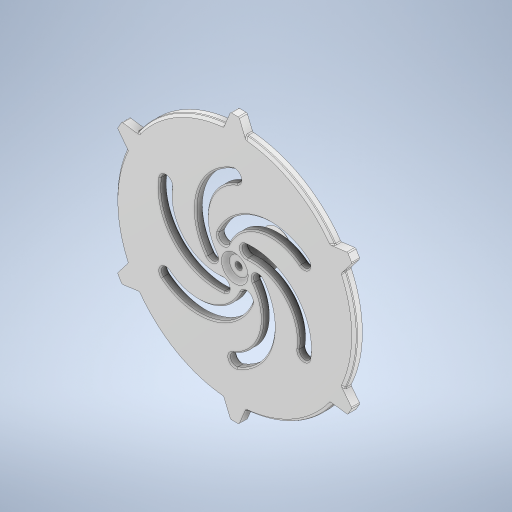
# Autodesk Inventor part: Spool Holder Iris Rotor
Saved by Autodesk Inventor 2024 (Build 280153000, 153)
## iProperties
Created: 2024-08-17
Part Number: Spool Holder Iris Rotor
Material: ABS Plastic
Document SubType Name: Modeling
Designer: Ishaan
Density: 1.06 g/cm^3
Appearance: Smooth - White
Author: Ishaan
Autodesk Inventor part; units mm, degrees
sketch "Sketch1" plane through (0, 0, 0) normal (0, 0, 1) x (1, 0, 0)
  circle A0 centre (0, 0) radius 90
  circle A1 centre (0, 0) radius 7
  dimension "d0" = 180
  dimension "d1" = 14
  constraints: 2 centre point, 2 coincident
  measures "d0" diameter of A0
  measures "d1" diameter of A1
extrude "Extrusion1" add sketch "Sketch1" against normal blind 6
sketch "Sketch2" plane through (0, 0, -6) normal (0, 0, -1) x (-1, 0, 0)
  circle A0 centre (0, 0) radius 90 projected
  circle A1 centre (0, 0) radius 7 projected
  circle A2 centre (0, 0) radius 9.9
  circle A3 centre (0, 0) radius 11
  dimension "d4" = 19.8
  dimension "d21" = 22
  constraints: 2 centre point, 2 coincident
  measures "d4" diameter of A2
  measures "d21" diameter of A3
extrude "Extrusion2" add sketch "Sketch2" along normal blind 16.4 contours A2 | A3
ref_plane "Work Plane1" through (0, 0, -26.65) normal (0, 0, -1) x (-1, 0, 0)
extrude "Extrusion3" add sketch "Sketch2" along normal up to surface (20.65 mm away) contours A2
ref_plane "Work Plane2" through (0, 0, -3) normal (0, 0, 1) x (1, 0, 0)
sketch "Sketch5" plane through (0, 0, -3) normal (0, 0, 1) x (1, 0, 0)
  circle A0 centre (0, 0) radius 7 projected
  circle A1 centre (0, 0) radius 90 projected
extrude "Extrusion6" add sketch "Sketch5" against normal up to surface (23.65 mm away) contours A0
chamfer "Chamfer8" distance 3 angle 45 1 edges at (-7, 0, 0)
chamfer "Chamfer4" distance 1 angle 45 1 edges at (11, 0, -6)
sketch "Sketch4" plane through (0, 0, 0) normal (0, 0, 1) x (1, 0, 0)
  circle A0 centre (-17.5, 0) radius 4.25 construction
  circle A1 centre (0, 0) radius 12 construction
  circle A2 centre (0, 60) radius 4.25 construction
  arc A3 (0, 60) -> (-17.5, 0) centre (14.0487, 23.3504) ccw construction
  arc A4 (-1.5212, 63.9684) -> (-20.9161, -2.5284) centre (14.0487, 23.3504) ccw
  arc A5 (1.5212, 56.0316) -> (-14.0839, 2.5284) centre (14.0487, 23.3504) ccw
  arc A6 (1.5212, 56.0316) -> (-1.5212, 63.9684) centre (0, 60) ccw
  arc A7 (-20.9161, -2.5284) -> (-14.0839, 2.5284) centre (-17.5, 0) ccw
  dimension "d32" = 8.5
  dimension "d33" = 17.5
  dimension "d35" = 60
  dimension "d36" = 35
  constraints: 10 point on circle, 7 centre point, 5 tangent, 1 equal radius, 1 horizontal alignment, 1 vertical alignment
  measures "d32" diameter of A0
  measures "d33" distance of point (0, 0) A0.centre
  measures "d35" distance of A2.centre point (0, 0)
  measures "d36" radius of A5
extrude "Extrusion5" cut sketch "Sketch4" against normal through all
pattern_circular "Circular Pattern1" count 6 over 360 about axis through (0, 0, 0) along (0, 0, -1) of "Extrusion5"
chamfer "Chamfer6" distance 2 angle 45 1 edges at (-90, 0, 0)
chamfer "Chamfer7" distance 1 angle 45 48 edges at (-38.4847, -0.3567, 0) (-4.5274, -14.6739, 0) (-44.6258, -6.2335, 0) (-51.2947, 34.1974, 0) (-38.4847, -0.3567, -6) (-51.2947, 34.1974, -6) (-44.6258, -6.2335, -6) (-4.5274, -14.6739, -6) (-18.9334, -33.5071, 0) (10.4442, -11.2577, 0) (-16.9146, -41.7638, 0) (-55.2631, -27.3238, 0) (-18.9334, -33.5071, -6) (-55.2631, -27.3238, -6) (-16.9146, -41.7638, -6) (10.4442, -11.2577, -6) (19.5513, -33.1504, 0) (14.9716, 3.4161, 0) (27.7113, -35.5304, 0) (-3.9684, -61.5212, 0) (19.5513, -33.1504, -6) (-3.9684, -61.5212, -6) (27.7113, -35.5304, -6) (14.9716, 3.4161, -6) (38.4847, 0.3567, 0) (4.5274, 14.6739, 0) (44.6258, 6.2335, 0) (51.2947, -34.1974, 0) (38.4847, 0.3567, -6) (51.2947, -34.1974, -6) (44.6258, 6.2335, -6) (4.5274, 14.6739, -6) (18.9334, 33.5071, 0) (-10.4442, 11.2577, 0) (16.9146, 41.7638, 0) (55.2631, 27.3238, 0) (18.9334, 33.5071, -6) (55.2631, 27.3238, -6) (16.9146, 41.7638, -6) (-10.4442, 11.2577, -6) (-19.5513, 33.1504, -6) (3.9684, 61.5212, -6) (-27.7113, 35.5304, -6) (-14.9716, -3.4161, -6) (-19.5513, 33.1504, 0) (-14.9716, -3.4161, 0) (-27.7113, 35.5304, 0) (3.9684, 61.5212, 0)
sketch "Sketch6" plane through (0, 0, -26.65) normal (0, 0, -1) x (-1, 0, 0)
  circle A0 centre (0, 0) radius 11 projected
extrude "Extrusion7" add sketch "Sketch6" along normal blind 6
chamfer "Chamfer9" distance 1 angle 45 1 edges at (11, 0, -32.65)
sketch "Sketch7" plane through (0, 0, -32.65) normal (0, 0, -1) x (-1, 0, 0)
  line L0 (0, -4.7631) -> (-4.125, -2.3816)
  line L1 (-4.125, -2.3816) -> (-4.125, 2.3816)
  line L2 (-4.125, 2.3816) -> (0, 4.7631)
  line L3 (0, 4.7631) -> (4.125, 2.3816)
  line L4 (4.125, 2.3816) -> (4.125, -2.3816)
  line L5 (4.125, -2.3816) -> (0, -4.7631)
  point P0 (0, 0)
  point P1 (0, 0)
  dimension "d59" = 8.25
  constraints: 12 end point, 1 coincident, 1 vertical, 13 other
  measures "d59" distance between parallel lines of L1 L4
extrude "Extrusion8" cut sketch "Sketch7" against normal blind 6
sketch "Sketch8" plane through (0, 0, -3) normal (0, 0, 1) x (1, 0, 0)
  circle A0 centre (0, 0) radius 11 projected
  constraints: 1 coincident
hole "Hole1" at (0, 0, -3) direction (0, 0, -1) diameter 5.3 end through all
ref_plane "Work Plane3" through (0, 0, -24.525) normal (0, 0, -1) x (-1, 0, 0)
split body "Split1" result two bodies by plane through (0, 0, -24.525) normal (0, 0, -1) first body at (-10.364, -1.6843, -29.9833)
sketch "Sketch9" plane through (0, 0, 0) normal (0, 0, 1) x (1, 0, 0)
  circle A0 centre (0, 0) radius 90 projected
  line L0 (7.5, -100) -> (-7.5, -100)
  line L1 (-7.5, -100) -> (-7.5, -80) construction
  line L2 (-7.5, -80) -> (7.5, -80) construction
  line L3 (7.5, -80) -> (7.5, -100) construction
  line L4 (7.5, -100) -> (-7.5, -80) construction
  line L5 (-7.5, -100) -> (7.5, -80) construction
  line L6 (-3.2282, -100) -> (-8.3638, -87.6016)
  line L7 (-8.3638, -87.6016) -> (8.3638, -87.6016)
  line L8 (8.3638, -87.6016) -> (3.2282, -100)
  circle A1 centre (0, 0) radius 88 construction
  line L9 (-3.2282, -100) -> (3.2282, -100) construction
  point P0 (0, -90)
  point P1 (0, -100)
  point P2 (-7.5, -89.687)
  point P3 (7.5, -89.687)
  dimension "d69" = 15
  dimension "d70" = 20
  dimension "d71" = 45
  constraints: 20 end point, 5 point on circle, 5 point on line, 4 midpoint, 3 horizontal, 2 parallel, 1 perpendicular, 1 vertical alignment
  measures "d69" distance of L1.end L2.end
  measures "d70" distance of L0.end L1.end
  measures "d71" angle of L8 L6
extrude "Extrusion9" add sketch "Sketch9" against normal up to surface (6 mm away) contours L6 L7 L8 A0 | A0 L8 L0 L6 picked at (-0.8342, -88.3895) bodies 3
fillet "Fillet2" radius 1 1 edges at (0, 90, -2)
pattern_circular "Circular Pattern2" count 6 over 360 about axis through (0, 0, -1.5) along (0, 0, 1) of "Extrusion9" bodies 3
fillet "Fillet3" radius 1 8 edges at (7.5328, -89.6078, -2.0315) (7.5, -89.687, -4.2071) (7.9967, -88.4877, -0.8483) (-7.5328, -89.6078, -2.0315) (-7.5, -89.687, -4.2071) (-7.9967, -88.4877, -0.8483) (-3.2282, -100, -3) (3.2282, -100, -3)
pattern_circular "Circular Pattern3" count 6 over 360 about axis through (0, 0, -1.5) along (0, 0, 1) of "Fillet3"
body "Solid2"
body "Solid3"
